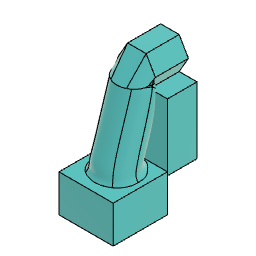
square to hex (Autodesk Fusion 360 design; units mm, degrees)
Autodesk Fusion 360 part; units mm, degrees
sketch "Sketch1" plane through (0, 0, 0) normal (0, 0, 1) x (1, 0, 0)
  line L0 (6, 6) -> (-6, 6)
  line L1 (-6, 6) -> (-6, -6)
  line L2 (-6, -6) -> (6, -6)
  line L3 (6, -6) -> (6, 6)
  line L4 (6, 6) -> (-6, -6) construction
  line L5 (-6, 6) -> (6, -6) construction
  line L6 (-11, 11) -> (11, 11)
  line L7 (11, 11) -> (11, -11)
  line L8 (11, -11) -> (-11, -11)
  line L9 (-11, -11) -> (-11, 11)
  line L10 (-11, 11) -> (11, -11) construction
  line L11 (11, 11) -> (-11, -11) construction
  dimension "d1" = 12
  dimension "d2" = 12
  dimension "d3" = 5
  constraint horizontal L0
  constraint perpendicular L0 L1
  constraint parallel L0 L2
  constraint parallel L1 L3
  constraint coincident L4 origin
  constraint coincident L5 origin
  constraint horizontal L6
  constraint perpendicular L6 L7
  constraint parallel L6 L8
  constraint parallel L7 L9
  constraint coincident L10 origin
  constraint coincident L11 origin
  constraint parallel L5 L10
  measures "d1" distance of L1.end L2.end
  measures "d2" distance of L0.end L1.end
  measures "d3" distance of L3 L7
extrude "Extrude1" add sketch "Sketch1" against normal blind 11.7 makes body 1
extrude "Extrude2" add sketch "Sketch1" along normal blind 2 contours L0 L1 L2 L3 | L6 L7 L8 L9 bodies 1
ref_plane "WorkPlane2" through (0, 11, 2) normal (0, 1, 0) x (-1, 0, 0)
sketch "Sketch3" plane through (0, 11, 0) normal (0, 1, 0) x (-1, 0, 0)
  line L0 (-3.7528, 31.5) -> (-7.5056, 25)
  line L1 (-7.5056, 25) -> (-3.7528, 18.5)
  line L2 (-3.7528, 18.5) -> (3.7528, 18.5)
  line L3 (3.7528, 18.5) -> (7.5056, 25)
  line L4 (7.5056, 25) -> (3.7528, 31.5)
  line L5 (3.7528, 31.5) -> (-3.7528, 31.5)
  line L6 (-11, 2) -> (11, 2)
  point P0 (0, 25)
  dimension "d10" = 13
  dimension "d19" = 16.5
  constraint horizontal L5
  measures "d10" distance of L2 L5
  measures "d19" distance of L2 L6
extrude "Extrude4" add sketch "Sketch3" along normal blind 12 separate body makes body 2
extrude "Extrude7" add 1 faces at (-3.6667, 3.6667, 2) along direction (0, 0, 1) up to surface (29.5 mm away) on bodies 1 bodies 1 2
chamfer "Chamfer2" distance 30.765 distance2 4.087 2 edges at (11, 0, 31.5) (-11, 0, 31.5) measured on face at (11, 3.6667, 2.7) measured on face at (-11, -3.6667, 17.1) on bodies 1
chamfer "Chamfer2" distance 30.506 distance2 13.341 1 edges at (0, -11, 31.5) measured on face at (3.6667, -11, 2.7) on bodies 1
fillet "Fillet2" radius 3.625 2 edges at (8.9393, -4.3295, 16.247) (-8.9393, -4.3295, 16.247) on bodies 1
equation "d19 = ( ( 27 / 2 ) * 1 mm ) + 3 mm"
